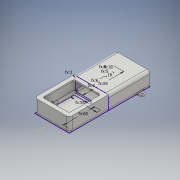
# Autodesk Inventor part: LED box
Saved by Autodesk Inventor 2018.3 (Build 223285000, 285)
## iProperties
Created: 2019-07-19
Part Number: LED box
Material: Generic
Document SubType Name: Modeling
Designer: uqspowe6
Density: 1 g/cm^3
Appearance: Default
wall_t: 3.000 mm
fillet_interior: 3.000 mm
fillet_exterior: 6.000 mm
opening_w: 65.000 mm
opening_h: 25.000 mm
window_w: 55.000 mm
window_h: 65.000 mm
seal_w: 8.000 mm
extension_h: 85.000 mm
mount_y: 20.000 mm
mount_dia: 8.000 mm
mount_hole: 3.200 mm
mount_x: 5.000 mm
Author: uqspowe6
Autodesk Inventor part; units mm, degrees
ref_plane "YZ Plane" through (0, 0, 0) normal (1, 0, 0) x (0, 1, 0)
ref_plane "XZ Plane" through (0, 0, 0) normal (0, 1, 0) x (-1, 0, 0)
ref_plane "XY Plane" through (0, 0, 0) normal (0, 0, 1) x (1, 0, 0)
sketch "Sketch1" plane through (0, 0, 0) normal (0, 0, 1) x (1, 0, 0)
  line L0 (-27.5, 32.5) -> (27.5, 32.5)
  line L1 (27.5, 32.5) -> (27.5, -32.5)
  line L2 (27.5, -32.5) -> (-27.5, -32.5)
  line L3 (-27.5, -32.5) -> (-27.5, 32.5)
  line L4 (-60.5, 0) -> (51.5, 0) construction
  line L5 (0, -73.7) -> (0, 158.7) construction
  line L6 (32.5, 37.5) -> (-32.5, 37.5)
  line L7 (-32.5, 37.5) -> (-32.5, -37.5)
  line L8 (-32.5, -37.5) -> (32.5, -37.5)
  line L9 (32.5, -37.5) -> (32.5, 37.5)
  line L10 (-35.5, -40.5) -> (-35.5, 40.5)
  line L11 (-35.5, 40.5) -> (35.5, 40.5)
  line L12 (35.5, 40.5) -> (35.5, -40.5)
  line L13 (35.5, -40.5) -> (-35.5, -40.5)
  line L14 (-35.5, 40.5) -> (-35.5, 125.5)
  line L15 (-35.5, 125.5) -> (35.5, 125.5)
  line L16 (35.5, 125.5) -> (35.5, 40.5)
  arc A0 (-41.7973, 101.7162) -> (-41.7973, 109.2838) centre (-40.5, 105.5) ccw construction
  line L17 (-29.5, 97.5) -> (-41.7973, 101.7162)
  line L18 (-41.7973, 109.2838) -> (-29.5, 113.5)
  arc A1 (-41.7973, 109.2838) -> (-41.7973, 101.7162) centre (-40.5, 105.5) ccw
  line L19 (-29.5, 97.5) -> (-29.5, 113.5)
  point P0 (0, 0)
  point P1 (-35.5, 99.5571)
  point P2 (-35.5, 111.4429)
  dimension "d0" = 55
  dimension "d1" = 65
  dimension "d2" = 5
  dimension "d6" = 3
  dimension "d33" = 85
  dimension "d34" = 8
  dimension "d39" = 6
  dimension "d40" = 16
  dimension "d41" = 20
  dimension "d50" = 5
  constraints: 38 end point, 6 parallel, 6 perpendicular, 4 point on circle, 4 point on line, 2 centre point, 2 tangent, 1 coincident, 1 equal length, 1 horizontal, 1 vertical, 8 other
  measures "d0" distance of L0.start L0.end
  measures "d1" distance of L0.end L1.end
  measures "d2" distance between parallel lines of L0 L6
  measures "d6" distance between parallel lines of L7 L10
  measures "d33" distance of L10.end L14.end
  measures "d34" diameter of A0
  measures "d39" distance between parallel lines of L19 L14
  measures "d40" distance of L18.end L17.start
  measures "d41" vertical distance of L14.end A0.centre
  measures "d50" distance from line of L14 A0.centre
extrude "Extrusion1" add sketch "Sketch1" against normal blind 3 contours L0 L1 L2 L3 | L9 L8 L7 L6 | L10 L11 L12 L13
extrude "Extrusion6" add sketch "Sketch1" along normal blind 25 contours L10 L11 L12 L13
sketch "Sketch2" plane through (0, 0, 25) normal (0, 0, 1) x (1, 0, 0)
  line L0 (32.5, 37.5) -> (32.5, -37.5) construction
  line L1 (32.5, -37.5) -> (-32.5, -37.5) construction
  line L2 (-32.5, -37.5) -> (-32.5, 37.5) construction
  line L3 (-32.5, 37.5) -> (32.5, 37.5) construction
  line L4 (-35.5, 40.5) -> (-35.5, -40.5) projected
  line L5 (-35.5, -40.5) -> (35.5, -40.5) projected
  line L6 (35.5, -40.5) -> (35.5, 40.5) projected
  line L7 (35.5, 40.5) -> (-35.5, 40.5) projected
  line L8 (-27.5, 32.5) -> (-27.5, -32.5)
  line L9 (-27.5, -32.5) -> (27.5, -32.5)
  line L10 (27.5, -32.5) -> (27.5, 32.5)
  line L11 (27.5, 32.5) -> (-27.5, 32.5)
  point P0 (0, 0)
  dimension "d20" = 5
  constraints: 8 end point, 3 other
  measures "d20" distance between parallel lines of L2 L8
extrude "Extrusion7" add sketch "Sketch2" along normal blind 3
sketch "Sketch3" plane through (-35.5, 40.5, -3) normal (0, 1, 0) x (1, 0, 0)
  line L0 (71, -31) -> (71, 0) construction
  line L1 (0, 0) -> (71, 0) construction
  line L2 (0, -31) -> (0, 0) construction
  line L3 (71, -31) -> (0, -31) construction
  line L4 (3, -25) -> (3, -6)
  line L5 (6, -3) -> (65, -3)
  line L6 (68, -6) -> (68, -25)
  line L7 (65, -28) -> (6, -28)
  arc A0 (3, -25) -> (6, -28) centre (6, -25) ccw
  arc A1 (6, -3) -> (3, -6) centre (6, -6) ccw
  arc A2 (68, -6) -> (65, -3) centre (65, -6) ccw
  arc A3 (65, -28) -> (68, -25) centre (65, -25) ccw
  line L8 (0, 0) -> (0, -31) construction
  line L9 (6, -31) -> (65, -31)
  line L10 (71, -25) -> (71, -6)
  line L11 (65, 0) -> (6, 0)
  line L12 (0, -6) -> (0, -25)
  arc A4 (0, -25) -> (6, -31) centre (6, -25) ccw
  arc A5 (6, 0) -> (0, -6) centre (6, -6) ccw
  arc A6 (71, -6) -> (65, 0) centre (65, -6) ccw
  arc A7 (65, -31) -> (71, -25) centre (65, -25) ccw
  point P0 (35.5, -3)
  point P1 (3, -28)
  point P2 (3, -3)
  point P3 (68, -3)
  point P4 (68, -28)
  dimension "d23" = 3
  dimension "d31" = 3
  constraints: 16 end point, 16 point on circle, 16 tangent, 12 point on line, 8 centre point, 6 equal radius, 2 parallel, 1 concentric, 1 horizontal, 1 perpendicular, 3 other
  measures "d23" distance between parallel lines of L3 L7
  measures "d31" radius of A0
extrude "Extrusion8" cut sketch "Sketch3" against normal up to next contours L4 A1 L5 A2 L6 A3 L7 A0
extrude "Extrusion9" add sketch "Sketch3" along normal up to surface (85 mm away)
fillet "Fillet1" radius 3 8 edges at (-32.5, 0, 25) (-32.5, 0, 0) (0, -37.5, 0) (0, -37.5, 25) (32.5, 0, 25) (-32.5, -37.5, 12.5) (32.5, -37.5, 12.5) (32.5, 0, 0)
fillet "Fillet1" radius 6 5 edges at (-35.5, -40.5, 12.5) (35.5, -40.5, 12.5) (0, -40.5, -3) (-35.5, 0, -3) (35.5, 0, -3)
fillet "Fillet1" radius 4 4 edges at (-27.5, -32.5, 26.5) (27.5, -32.5, 26.5) (27.5, 32.5, 26.5) (-27.5, 32.5, 26.5)
extrude "Extrusion10" add sketch "Sketch1" against normal blind 3 contours L17 A1 L18 L14 | L14 L18 L19 L17
hole "Hole1" at (-40.5, 105.5, 0) direction (0, 0, -1) diameter 3.2 end through all
mirror "Mirror1" about plane through (0, 0, 0) normal (1, 0, 0) of "Hole1", "Extrusion10"
fillet "Fillet2" radius 3 4 edges at (-32.5, 112.4714, -2.1962) (-32.5, 98.5286, -2.1962) (32.5, 112.4714, -2.1962) (32.5, 98.5286, -2.1962)
fillet "Fillet2" radius 1 2 edges at (-34.6962, 105.5, 0) (34.6962, 105.5, 0)
equation "\"d0\" = window_w"
equation "\"d1\" = window_h"
equation "\"d2\" = seal_w - wall_t"
equation "\"d6\" = wall_t"
equation "\"d33\" = extension_h"
equation "\"d34\" = mount_dia"
equation "\"d39\" = fillet_exterior"
equation "\"d41\" = mount_y"
equation "\"d50\" = mount_x"
equation "\"d18\" = opening_h"
equation "\"d20\" = d2"
equation "\"d23\" = wall_t"
equation "\"d31\" = fillet_interior"
equation "\"d42\" = mount_hole"
equation "\"window_w\" = 55"
equation "\"window_h\" = 65"
equation "\"wall_t\" = 3"
equation "\"seal_w\" = 8"
equation "\"extension_h\" = 85"
equation "\"mount_y\" = 20"
equation "\"mount_dia\" = 8"
equation "\"mount_hole\" = 3.2"
equation "\"fillet_interior\" = 3"
equation "\"fillet_exterior\" = fillet_interior + wall_t"
equation "\"mount_x\" = 5"
equation "\"opening_w\" = window_w + 2 * seal_w - 2 * wall_t"
equation "\"opening_h\" = 25"
body "Solid1"
